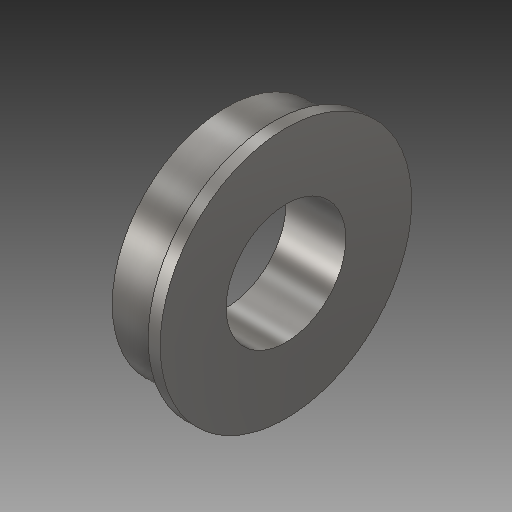
# Autodesk Inventor part: F688ZZ 8mm ID Flange
Saved by Autodesk Inventor 2019 (Build 230136000, 136)
## iProperties
Created: 2019-10-19
Part Number: F688ZZ 8mm ID Flange
Material: Stainless Steel
Document SubType Name: Modeling
Designer: admin
Density: 8 g/cm^3
Appearance: Semi-Polished
Author: admin
Autodesk Inventor part; units mm, degrees
ref_plane "YZ Plane" through (0, 0, 0) normal (1, 0, 0) x (0, 1, 0)
ref_plane "XZ Plane" through (0, 0, 0) normal (0, 1, 0) x (-1, 0, 0)
ref_plane "XY Plane" through (0, 0, 0) normal (0, 0, 1) x (1, 0, 0)
sketch "Sketch1" plane through (0, 0, 0) normal (0, 0, 1) x (1, 0, 0)
  line L0 (0, 9.5) -> (0, 5)
  line L1 (0, 5) -> (5, 5)
  line L2 (5, 5) -> (5, 10.5)
  line L3 (5, 10.5) -> (4, 10.5)
  line L4 (4, 10.5) -> (4, 9.5)
  line L5 (4, 9.5) -> (0, 9.5)
  line L6 (0, 0) -> (4.5572, 0) construction
  dimension "d0" = 5
  dimension "d1" = 9.5
  dimension "d2" = 1
  dimension "d3" = 5
  dimension "d4" = 10.5
  constraints: 14 end point, 5 perpendicular, 1 horizontal, 1 point on line, 1 vertical
  measures "d0" distance from line of L6.start L1
  measures "d1" distance from line of L6.start L5
  measures "d2" distance of L2.end L3.end
  measures "d3" distance between parallel lines of L2 L0
  measures "d4" distance from line of L6.start L3
revolve "Revolution1" add sketch "Sketch1" angle 360 about axis through (0, 0, 0) along (1, 0, 0)
body "Solid1"
